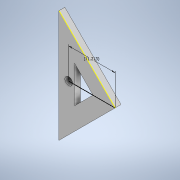
# Autodesk Inventor part: Eslabon_3_inventor
Saved by Autodesk Inventor 2021 (Build 250183000, 183)
## iProperties
Created: 2021-08-13
Part Number: Eslabon_3_inventor
Material: Genérico
Document SubType Name: Modeling
Designer: uriel
Density: 1 g/cm^3
Appearance: Valor por defecto
Author: uriel
Autodesk Inventor part; units mm, degrees
ref_plane "YZ Plane" through (0, 0, 0) normal (1, 0, 0) x (0, 1, 0)
ref_plane "XZ Plane" through (0, 0, 0) normal (0, 1, 0) x (-1, 0, 0)
ref_plane "XY Plane" through (0, 0, 0) normal (0, 0, 1) x (1, 0, 0)
sketch "Boceto1" plane through (0, 0, 0) normal (0, 0, 1) x (1, 0, 0)
  circle A0 centre (0, 0) radius 6
  line L0 (0, 0) -> (0, 50)
  line L1 (0, 0) -> (50, 0)
  line L2 (50, 0) -> (0, 50)
  line L3 (0, 0) -> (0, -50)
  line L4 (0, -50) -> (50, 0)
  line L5 (60.6066, 10.6066) -> (-15, 86.2132)
  line L6 (-15, 86.2132) -> (-15, 0)
  line L7 (60.6066, -10.6066) -> (-15, -86.2132)
  line L8 (-15, -86.2132) -> (-15, 0)
  line L9 (60.6066, -10.6066) -> (71.2132, 0)
  line L10 (71.2132, 0) -> (60.6066, 10.6066)
  line L11 (9, 0) -> (9, 28.2721)
  line L12 (9, 28.2721) -> (43.636, -6.364)
  line L13 (43.636, 6.364) -> (9, -28.2721)
  line L14 (9, -28.2721) -> (9, 0)
  point P0 (37.2721, 0)
  dimension "d0" = 12
  dimension "d1" = 50
  dimension "d2" = 50
  dimension "d3" = 50
  dimension "d4" = 15
  dimension "d5" = 15
  dimension "d6" = 9
  dimension "d7" = 9
  constraints: 30 end point, 3 perpendicular, 1 centre point, 1 coincident, 1 parallel, 1 vertical, 4 other
  measures "d0" diameter of A0
  measures "d1" distance of L0.start L0.end
  measures "d2" distance of L0.start L1.end
  measures "d3" distance of L0.start L3.end
  measures "d4" distance between parallel lines of L2 L5
  measures "d5" distance between parallel lines of L4 L7
  measures "d6" distance between parallel lines of L0 L11
  measures "d7" distance between parallel lines of L4 L13
extrude "Extrusión1" add sketch "Boceto1" along normal blind 9 contours L1 L14 L13 L12 L4 L3 A0 | A0 L0 L2 L13 L12 L11 L1 | L13 L2 L1 | L1 L4 L12 | L10 L9 L7 L8 L6 L5
sketch "Boceto2" plane through (0, 0, 9) normal (0, 0, 1) x (1, 0, 0)
  line L0 (71.2132, 0) -> (-15, 86.2132) projected
  line L1 (0, 0) -> (71.2132, 0)
  dimension "d10" = 71.2132
  constraints: 2 end point, 1 horizontal
  measures "d10" distance of L1.start L0.start
equation "\"d8\" = d7"
